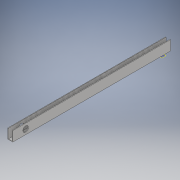
# Autodesk Inventor part: 36in Aluminum Channel
Saved by Autodesk Inventor 2018 (Build 220112000, 112)
## iProperties
Created: 2019-01-13
Part Number: 36in Aluminum Channel
Material: Generic
Document SubType Name: Modeling
Designer: Gabriel
Density: 1 g/cm^3
Appearance: Default
Author: Gabriel
Autodesk Inventor part; units mm, degrees
ref_plane "YZ Plane" through (0, 0, 0) normal (1, 0, 0) x (0, 1, 0)
ref_plane "XZ Plane" through (0, 0, 0) normal (0, 1, 0) x (-1, 0, 0)
ref_plane "XY Plane" through (0, 0, 0) normal (0, 0, 1) x (1, 0, 0)
sketch "Sketch1" plane through (0, 0, 0) normal (0, 1, 0) x (-1, 0, 0)
  line L0 (23.5034, -42.4981) -> (-1.8966, -42.4981)
  line L1 (-1.8966, -42.4981) -> (-1.8966, 770.3019)
  line L2 (-1.8966, 770.3019) -> (23.5034, 770.3019)
  line L3 (23.5034, 770.3019) -> (23.5034, -42.4981)
  line L4 (20.3284, -39.3231) -> (1.2784, -39.3231)
  line L5 (1.2784, -39.3231) -> (1.2784, 767.1269)
  line L6 (1.2784, 767.1269) -> (20.3284, 767.1269)
  line L7 (20.3284, 767.1269) -> (20.3284, -39.3231)
  point P0 (0, 0)
  dimension "d0" = 25.4
  dimension "d1" = 812.8
  dimension "d2" = 3.175
  constraints: 16 end point, 4 parallel, 2 perpendicular, 1 horizontal, 3 other
  measures "d0" distance of L1.end L2.end
  measures "d1" distance of L0.end L1.end
  measures "d2" distance between parallel lines of L3 L7
ref_plane "Work Plane3" through (0, 0, 0) normal (0, -1, 0) x (1, 0, 0)
sketch "Sketch2" plane through (0, 0, 0) normal (0, -1, 0) x (1, 0, 0)
  line L0 (-1.2784, -39.3231) -> (-20.3284, -39.3231) projected
  line L1 (-20.3284, -39.3231) -> (-20.3284, 767.1269) projected
  line L2 (-1.2784, -39.3231) -> (-20.3284, -39.3231)
  line L3 (-20.3284, -39.3231) -> (-20.3284, 767.1269)
  line L4 (-20.3284, 767.1269) -> (-1.2784, 767.1269)
  line L5 (-1.2784, 767.1269) -> (-1.2784, -39.3231)
  point P0 (0, 0)
  constraints: 8 end point, 2 parallel, 1 horizontal, 1 perpendicular
extrude "Extrusion3" add sketch "Sketch2" against normal blind 3.175
extrude "Extrusion5" add sketch "Sketch1" along normal blind 50.8
sketch "Sketch4" plane through (-23.5034, 0, 770.3019) normal (0, 0, 1) x (1, 0, 0)
  line L0 (0, 50.8) -> (25.4, 50.8) projected
  line L1 (0, 50.8) -> (3.175, 50.8)
  line L2 (3.175, 50.8) -> (25.4, 50.8)
  line L3 (25.4, 50.8) -> (22.225, 50.8)
  line L4 (22.225, 3.175) -> (22.225, 50.8) projected
  line L5 (3.175, 50.8) -> (22.225, 50.8)
  line L6 (22.225, 50.8) -> (22.225, 3.175)
  line L7 (22.225, 3.175) -> (3.175, 3.175)
  line L8 (3.175, 3.175) -> (3.175, 50.8)
  point P0 (23.5034, 0)
  point P1 (22.225, 0)
  dimension "d13" = 3.175
  dimension "d14" = 3.175
  constraints: 14 end point, 2 parallel, 2 point on line, 1 collinear, 1 horizontal, 1 perpendicular
  measures "d13" distance of L0.start L1.end
  measures "d14" distance of L0.end L3.end
extrude "Extrusion6" cut sketch "Sketch4" against normal blind 1016
sketch "Sketch5" plane through (1.8966, 0, 770.3019) normal (1, 0, 0) x (0, 0, -1)
  line L0 (0, 0) -> (66.04, 0)
  line L1 (66.04, 0) -> (66.04, 25.4)
  line L2 (66.04, 25.4) -> (0, 25.4)
  line L3 (0, 25.4) -> (0, 0)
  circle A0 centre (66.04, 25.4) radius 14.2875
  point P0 (770.3019, 0)
  dimension "d17" = 66.04
  dimension "d18" = 25.4
  dimension "d19" = 28.575
  constraints: 8 end point, 2 parallel, 1 centre point, 1 coincident, 1 horizontal, 1 perpendicular
  measures "d17" distance of L2.end L1.end
  measures "d18" distance of L1.end L0.end
  measures "d19" diameter of A0
extrude "Extrusion7" cut sketch "Sketch5" against normal blind 1016 contours A0 L2 L1 | L1 L2 A0
body "Solid2"
